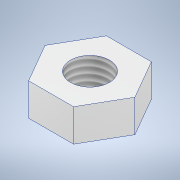
# Autodesk Inventor part: M3_nut_2,5mm
Saved by Autodesk Inventor 2020.3 (Build 243373000, 373)
## iProperties
Created: 2021-03-23
Part Number: M3_nut_2,5mm
Material: Aluminum 6061
Document SubType Name: Modeling
Designer: patry
Density: 2.7 g/cm^3
Appearance: Aluminum - Flat
Mass: 0.28647 g
Surface Area: 1.71754 cm^2
Volume: 0.1061 cm^3
Author: patry
Autodesk Inventor part; units mm, degrees
ref_plane "YZ Plane" through (0, 0, 0) normal (1, 0, 0) x (0, 1, 0)
ref_plane "XZ Plane" through (0, 0, 0) normal (0, 1, 0) x (-1, 0, 0)
ref_plane "XY Plane" through (0, 0, 0) normal (0, 0, 1) x (1, 0, 0)
sketch "Szkic1" plane through (0, 0, 0) normal (0, 1, 0) x (-1, 0, 0)
  line L0 (-1.7321, -3) -> (-3.4641, 0)
  line L1 (-3.4641, 0) -> (-1.7321, 3)
  line L2 (-1.7321, 3) -> (1.7321, 3)
  line L3 (1.7321, 3) -> (3.4641, 0)
  line L4 (3.4641, 0) -> (1.7321, -3)
  line L5 (1.7321, -3) -> (-1.7321, -3)
  circle A0 centre (0, 0) radius 1.5
  dimension "d0" = 6
  dimension "d1" = 3
  constraints: 12 end point, 2 coincident, 1 centre point, 13 other
  measures "d0" distance between parallel lines of L2 L5
  measures "d1" diameter of A0
extrude "Wyciągnięcie proste1" add sketch "Szkic1" along normal blind 2.5
thread "Gwint1" size "M3x0.5" class "6H" standard "ANSI Metric M Profile" length 5
